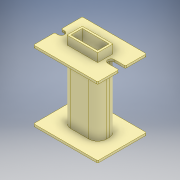
# Autodesk Inventor part: kicker_tube
Saved by Autodesk Inventor 2018 (Build 220112000, 112)
## iProperties
Created: 2019-01-25
Part Number: kicker_tube
Material: Nylon 6/6
Document SubType Name: Modeling
Designer: steve
Density: 1.13 g/cm^3
Appearance: Nylon 6
Author: steve
## iProperties of the stored document kicker_tube_3DPrint.ipt
Created: 2019-05-16
Part Number: kicker_tube_3DPrint
Material: Generic
Document SubType Name: Modeling
Designer: steve
Density: 1 g/cm^3
Appearance: Default
Author: steve
Autodesk Inventor part; units mm, degrees
ref_plane "YZ Plane" through (0, 0, 0) normal (1, 0, 0) x (0, 1, 0)
ref_plane "XZ Plane" through (0, 0, 0) normal (0, 1, 0) x (-1, 0, 0)
sketch "Sketch1" plane through (0, 0, 0) normal (0, 0, 1) x (1, 0, 0)
  line L0 (-6.075, -2.575) -> (6.075, -2.575)
  line L1 (6.075, -2.575) -> (6.075, 2.575)
  line L2 (6.075, 2.575) -> (-6.075, 2.575)
  line L3 (-6.075, 2.575) -> (-6.075, -2.575)
  line L4 (-6.075, -2.575) -> (6.075, 2.575) construction
  line L5 (6.075, -2.575) -> (-6.075, 2.575) construction
  line L6 (-8.075, 4.575) -> (8.075, 4.575)
  line L7 (8.075, 4.575) -> (8.075, -4.575)
  line L8 (8.075, -4.575) -> (-8.075, -4.575)
  line L9 (-8.075, -4.575) -> (-8.075, 4.575)
  point P0 (0, 0)
  dimension "d0" = 5.15
  dimension "d1" = 12.15
  dimension "d2" = 2
  constraints: 20 end point, 4 parallel, 2 midpoint, 2 perpendicular, 1 horizontal, 3 other
  measures "d0" distance between parallel lines of L0 L2
  measures "d1" distance between parallel lines of L1 L3
  measures "d2" distance between parallel lines of L2 L6
extrude "Extrusion1" add sketch "Sketch1" along normal blind 30
sketch "Sketch2" plane through (0, 0, 30) normal (0, 0, 1) x (1, 0, 0)
  line L0 (14.575, -11.075) -> (-14.575, -11.075)
  line L1 (-14.575, -11.075) -> (-14.575, 11.075)
  line L2 (-14.575, 11.075) -> (14.575, 11.075)
  line L3 (14.575, 11.075) -> (14.575, -11.075)
  line L4 (14.575, -11.075) -> (-14.575, 11.075) construction
  line L5 (-14.575, -11.075) -> (14.575, 11.075) construction
  line L6 (8.075, 4.575) -> (-8.075, 4.575) construction
  line L7 (-8.075, 4.575) -> (-8.075, -4.575) construction
  line L8 (8.075, -4.575) -> (8.075, 4.575) construction
  line L9 (-6.075, -2.575) -> (-6.075, 2.575) projected
  line L10 (-6.075, 2.575) -> (6.075, 2.575) projected
  line L11 (6.075, 2.575) -> (6.075, -2.575) projected
  line L12 (6.075, -2.575) -> (-6.075, -2.575) projected
  line L13 (8.075, 4.575) -> (-8.075, 4.575) projected
  line L14 (-8.075, 4.575) -> (-8.075, -4.575) projected
  line L15 (-8.075, -4.575) -> (8.075, -4.575) construction
  line L16 (8.075, -4.575) -> (8.075, 4.575) projected
  point P0 (0, 0)
  dimension "d5" = 6.5
  dimension "d6" = 6.5
  constraints: 12 end point, 2 midpoint, 2 parallel, 1 horizontal, 1 perpendicular
  measures "d5" distance between parallel lines of L2 L6
  measures "d6" distance between parallel lines of L7 L1
extrude "Extrusion2" add sketch "Sketch2" along normal blind 1
ref_plane "Work Plane1" through (0, 0, 15) normal (0, 0, -1) x (-1, 0, 0)
mirror "Mirror1" about plane through (0, 0, 15) normal (0, 0, -1) of "Extrusion2"
fillet "Fillet1" radius 4 4 edges at (8.075, 4.575, 15) (8.075, -4.575, 15) (-8.075, -4.575, 15) (-8.075, 4.575, 15)
sketch "Sketch3" plane through (0, 0, 31) normal (0, 0, 1) x (1, 0, 0)
  line L0 (6.075, 2.575) -> (6.075, -2.575) projected
  line L1 (-6.075, 2.575) -> (6.075, 2.575) projected
  line L2 (-6.075, -2.575) -> (-6.075, 2.575) projected
  line L3 (6.075, -2.575) -> (-6.075, -2.575) projected
  line L4 (-6.975, -3.475) -> (-6.975, 3.475)
  line L5 (-6.975, 3.475) -> (6.975, 3.475)
  line L6 (6.975, 3.475) -> (6.975, -3.475)
  line L7 (6.975, -3.475) -> (-6.975, -3.475)
  point P0 (0, 0)
  dimension "d10" = 0.9
  constraints: 8 end point, 3 other
  measures "d10" distance between parallel lines of L3 L7
extrude "Extrusion3" add sketch "Sketch3" along normal blind 3.9
mirror "Mirror2" about plane through (0, 0, 15) normal (0, 0, -1) of "Extrusion3"
sketch "Sketch5" plane through (0, 0, 30) normal (0, 0, -1) x (-1, 0, 0)
  line L0 (-8.075, -0.575) -> (-8.075, 0.575) construction
  line L1 (-20.405, 0) -> (20.405, 0) construction
  line L2 (-8.075, -1.5) -> (-14.575, -1.5) construction
  line L3 (-14.575, -1.5) -> (-14.575, 1.5) construction
  line L4 (-14.575, 1.5) -> (-8.075, 1.5) construction
  line L5 (-8.075, 1.5) -> (-8.075, -1.5) construction
  line L6 (-8.075, -1.5) -> (-14.575, 1.5) construction
  line L7 (-14.575, -1.5) -> (-8.075, 1.5) construction
  line L8 (-14.575, -11.075) -> (-14.575, 11.075) construction
  arc A0 (-9.575, -1.5) -> (-9.575, 1.5) centre (-9.575, 0) ccw
  line L9 (-9.575, 1.5) -> (-14.575, 1.5)
  line L10 (-14.575, 1.5) -> (-14.575, -1.5)
  line L11 (-14.575, -1.5) -> (-9.575, -1.5)
  line L12 (-9.575, 0) -> (-9.575, 1.9655) construction
  line L13 (11.575, 3.0291) -> (11.575, -4.4188) construction
  line L14 (14.575, 11.075) -> (14.575, -11.075) construction
  line L15 (14.575, -1.5) -> (11.575, -1.5) construction
  line L16 (11.575, -1.5) -> (11.575, 1.5) construction
  line L17 (11.575, 1.5) -> (14.575, 1.5) construction
  line L18 (14.575, 1.5) -> (14.575, -1.5) construction
  line L19 (14.575, -1.5) -> (11.575, 1.5) construction
  line L20 (11.575, -1.5) -> (14.575, 1.5) construction
  arc A1 (13.075, 1.5) -> (13.075, -1.5) centre (13.075, 0) ccw
  line L21 (13.075, 1.5) -> (14.575, 1.5)
  line L22 (14.575, 1.5) -> (14.575, -1.5)
  line L23 (14.575, -1.5) -> (13.075, -1.5)
  point P0 (0, 0)
  point P1 (-11.325, 0)
  dimension "d13" = 3
  dimension "d14" = 1.5
  dimension "d15" = 3
  dimension "d16" = 1.5
  dimension "d17" = 3
  constraints: 40 end point, 7 collinear, 7 point on line, 6 midpoint, 4 parallel, 4 point on circle, 3 perpendicular, 2 centre point, 2 coincident, 2 horizontal, 2 vertical
  measures "d13" distance between parallel lines of L2 L4
  measures "d14" distance from line of L5 point (-9.575, 0)
  measures "d15" distance between parallel lines of L13 L14
  measures "d16" distance from line of L13 point (13.075, 0)
  measures "d17" distance between parallel lines of L15 L17
extrude "Extrusion4" cut sketch "Sketch5" against normal through all
fillet "Fillet2" radius 0.5 12 edges at (14.575, 1.5, 30.5) (14.575, -1.5, 30.5) (-14.575, 1.5, 30.5) (-14.575, -1.5, 30.5) (-14.575, 11.075, 30.5) (14.575, 11.075, 30.5) (14.575, -11.075, 30.5) (-14.575, -11.075, 30.5) (-14.575, -11.075, -0.5) (-14.575, 11.075, -0.5) (14.575, 11.075, -0.5) (14.575, -11.075, -0.5)
equation "\"d2\" = ep"
equation "\"ep\" = 2"
body "Solid1"
